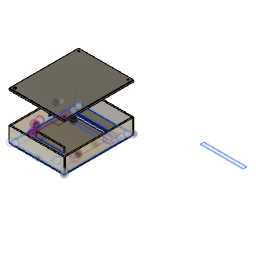
ArduinoCase v21 (Autodesk Fusion 360 design; units mm, degrees)
Autodesk Fusion 360 part; units mm, degrees
note: some values were not read from the file. Chosen so that the rebuilt part matches the saved one: which bodies a step acts on; which face or edge a step refers to; which pieces of a blend or face edit are solid. Set by a fixed rule: which sketch regions a step uses.
sketch "スケッチ1" plane through (0, 0, 0) normal (0, 0, 1) x (1, 0, 0)
  line L0 (0, 0) -> (66.06, 0)
  line L1 (68.6, 5.08) -> (68.6, 38.06)
  line L2 (64.79, 53.3) -> (0, 53.3)
  line L3 (0, 53.3) -> (0, 0)
  line L4 (64.79, 53.3) -> (68.6, 53.3)
  line L5 (68.6, 53.3) -> (68.6, 38.06)
  line L6 (66.06, 0) -> (68.6, 0)
  line L7 (68.6, 0) -> (68.6, 5.08)
  dimension "d6" = 68.6
  dimension "d7" = 53.3
  constraint horizontal L0
  constraint vertical L1
  constraint horizontal L2
  constraint vertical L3
  constraint coincident L0.start L3.end
  constraint perpendicular L1 L4
  constraint perpendicular L4 L5
  constraint perpendicular L1 L6
  constraint perpendicular L6 L7
  measures "d6" distance of L1 L3
  measures "d7" distance of L0.start L2.end
extrude "押し出し1" add sketch "スケッチ1" along normal blind 1.6 makes body 1
ref_plane "作業平面1" through (34.3, 26.65, 1.6) normal (0, 0, 1) x (1, 0, 0)
sketch "スケッチ2" plane through (34.3, 26.65, 1.6) normal (0, 0, 1) x (1, 0, 0)
  circle A0 centre (-20.33, -24.11) radius 1.6
  circle A1 centre (31.74, -19.03) radius 1.6
  circle A2 centre (31.74, 8.91) radius 1.6
  circle A3 centre (-19.06, 24.15) radius 1.6
  line L0 (-34.3, -26.65) -> (34.3, -26.65)
  line L1 (-34.3, 26.65) -> (-34.3, -26.65)
  dimension "d15" = 3.2
  dimension "d16" = 3.2
  dimension "d17" = 3.2
  dimension "d18" = 3.2
  dimension "d19" = 2.54
  dimension "d20" = 13.97
  dimension "d48" = 66.04
  dimension "d49" = 7.62
  dimension "d50" = 35.56
  dimension "d51" = 66.04
  dimension "d52" = 15.24
  dimension "d53" = 50.8
  measures "d15" diameter of A3
  measures "d16" diameter of A2
  measures "d17" diameter of A1
  measures "d18" diameter of A0
  measures "d19" distance of A0.centre L0
  measures "d20" distance of A0.centre L1
  measures "d48" distance of A1.centre L1
  measures "d49" distance of A1.centre L0
  measures "d50" distance of A2.centre L0
  measures "d51" distance of A2.centre L1
  measures "d52" distance of A3.centre L1
  measures "d53" distance of A3.centre L0
extrude "押し出し2" cut sketch "スケッチ2" against normal up to surface (1.6 mm away) bodies 1
sketch "スケッチ3" plane through (34.3, 26.65, 1.6) normal (0, 0, 1) x (1, 0, 0)
  line L0 (-36.1, -14.45) -> (-22.1, -14.45)
  line L1 (-22.1, -14.45) -> (-22.1, -23.35)
  line L2 (-22.1, -23.35) -> (-36.1, -23.35)
  line L3 (-36.1, -23.35) -> (-36.1, -14.45)
  line L4 (-34.3, 26.65) -> (-34.3, -26.65)
  line L5 (-34.3, -26.65) -> (34.3, -26.65)
  dimension "d28" = 8.9
  dimension "d29" = 14
  dimension "d30" = 1.8
  dimension "d31" = 3.3
  constraint horizontal L0
  constraint vertical L1
  constraint horizontal L2
  constraint vertical L3
  measures "d28" distance of L0.start L2.end
  measures "d29" distance of L0.start L0.end
  measures "d30" distance of L3 L4
  measures "d31" distance of L2 L5
extrude "押し出し3" add sketch "スケッチ3" along normal blind 10.9 separate body makes body 2
sketch "スケッチ4" plane through (34.3, 26.65, 1.6) normal (0, 0, 1) x (1, 0, 0)
  line L0 (-40.5, 17.05) -> (-24.5, 17.05)
  line L1 (-24.5, 17.05) -> (-24.5, 5.05)
  line L2 (-24.5, 5.05) -> (-40.5, 5.05)
  line L3 (-40.5, 5.05) -> (-40.5, 17.05)
  line L4 (34.3, 26.65) -> (-34.3, 26.65)
  line L5 (-34.3, 26.65) -> (-34.3, -26.65)
  dimension "d34" = 12
  dimension "d35" = 16
  dimension "d36" = 9.6
  dimension "d37" = 6.2
  constraint horizontal L0
  constraint vertical L1
  constraint horizontal L2
  constraint vertical L3
  measures "d34" distance of L0.start L2.end
  measures "d35" distance of L0.start L0.end
  measures "d36" distance of L0 L4
  measures "d37" distance of L3 L5
extrude "押し出し4" add sketch "スケッチ4" along normal blind 10.9 separate body makes body 3
shell "シェル1" thickness 1 removed faces 1 at (-6.2, 35.7, 5.2333) on bodies 3
ref_plane "作業平面2" through (-1.8, 7.75, 7.05) normal (-1, 0, 0) x (0, -1, 0)
sketch "スケッチ5" plane through (-1.8, 7.75, 7.05) normal (-1, 0, 0) x (0, 1, 0)
  circle A0 centre (0.05, -0.95) radius 4
  line L0 (4.45, -5.45) -> (-4.45, -5.45)
  line L1 (-4.45, 5.45) -> (-4.45, -5.45)
  dimension "d42" = 8
  dimension "d43" = 4.5
  dimension "d44" = 4.5
  measures "d42" diameter of A0
  measures "d43" distance of A0.centre L0
  measures "d44" distance of A0.centre L1
extrude "押し出し5" cut sketch "スケッチ5" against normal blind 12 bodies 2
sketch "Sketch13" plane through (0, 0, 1.6) normal (0, 0, 1) x (-1, 0, 0)
  circle A0 centre (-15.24, -50.8) radius 1.6
  circle A1 centre (-66.04, -35.56) radius 1.6
  circle A2 centre (-13.97, -2.54) radius 1.6
  circle A3 centre (-66.04, -7.62) radius 1.6
  line L0 (-68.6, -53.3) -> (0, -53.3)
  line L1 (0, -53.3) -> (0, 0)
  line L2 (0, 0) -> (-68.6, 0)
  line L3 (-68.6, 0) -> (-68.6, -53.3)
  line L4 (4.8948, -79.4441) -> (-81.6052, -79.4441)
  line L5 (-81.6052, -79.4441) -> (-81.6052, 30.5559)
  line L6 (-81.6052, 30.5559) -> (4.8948, 30.5559)
  line L7 (4.8948, 30.5559) -> (4.8948, -79.4441)
  line L8 (4.8948, -79.4441) -> (-2.1052, -79.4441)
  line L9 (-2.1052, -79.4441) -> (-2.1052, -80.4441)
  line L10 (5.8948, -72.4441) -> (4.8948, -72.4441)
  line L11 (4.8948, -72.4441) -> (4.8948, -79.4441)
  line L12 (-81.6052, -79.4441) -> (-74.6052, -79.4441)
  line L13 (-74.6052, -79.4441) -> (-74.6052, -80.4441)
  line L14 (-82.6052, -72.4441) -> (-81.6052, -72.4441)
  line L15 (-81.6052, -72.4441) -> (-81.6052, -79.4441)
  line L16 (4.8948, 30.5559) -> (-2.1052, 30.5559)
  line L17 (-2.1052, 30.5559) -> (-2.1052, 31.5559)
  line L18 (5.8948, 23.5559) -> (4.8948, 23.5559)
  line L19 (4.8948, 23.5559) -> (4.8948, 30.5559)
  line L20 (-81.6052, 30.5559) -> (-74.6052, 30.5559)
  line L21 (-74.6052, 30.5559) -> (-74.6052, 31.5559)
  line L22 (-82.6052, 23.5559) -> (-81.6052, 23.5559)
  line L23 (-81.6052, 23.5559) -> (-81.6052, 30.5559)
  arc A4 (5.8948, -72.4441) -> (-2.1052, -80.4441) centre (5.8948, -80.4441) ccw
  arc A5 (-74.6052, -80.4441) -> (-82.6052, -72.4441) centre (-82.6052, -80.4441) ccw
  arc A6 (-82.6052, 23.5559) -> (-74.6052, 31.5559) centre (-82.6052, 31.5559) ccw
  arc A7 (-2.1052, 31.5559) -> (5.8948, 23.5559) centre (5.8948, 31.5559) ccw
  line L24 (-4.5368, 3.1002) -> (-53.3368, 3.1002)
  line L25 (-53.3368, 3.1002) -> (-53.3368, 29.1002)
  line L26 (-53.3368, 29.1002) -> (-4.5368, 29.1002)
  line L27 (-4.5368, 29.1002) -> (-4.5368, 3.1002)
  line L28 (-53.3368, 3.1002) -> (-8.3368, 3.1002)
  line L29 (-8.3368, 3.1002) -> (-8.3368, 1.1002)
  line L30 (-8.3368, 1.1002) -> (-53.3368, 1.1002)
  line L31 (-53.3368, 1.1002) -> (-53.3368, 3.1002)
  line L32 (-152.4076, -126.3216) -> (-222.4076, -126.3216)
  line L33 (-222.4076, -126.3216) -> (-222.4076, -122.3216)
  line L34 (-222.4076, -122.3216) -> (-152.4076, -122.3216)
  line L35 (-152.4076, -122.3216) -> (-152.4076, -126.3216)
  circle A8 centre (2.0051, -76.5556) radius 1.85
  circle A9 centre (-78.6355, -76.6374) radius 1.85
  circle A10 centre (-78.6896, 27.6935) radius 1.85
  circle A11 centre (2.0228, 27.6497) radius 1.85
  circle A12 centre (-15.24, -50.8) radius 2.5
  circle A13 centre (-66.04, -7.62) radius 2.5
  line L36 (1.0324, -67.1894) -> (-78.9676, -67.1894)
  line L37 (-78.9676, -67.1894) -> (-78.9676, -47.1894)
  line L38 (-78.9676, -47.1894) -> (1.0324, -47.1894)
  line L39 (1.0324, -47.1894) -> (1.0324, -67.1894)
  line L40 (-72.9759, 3.4319) -> (-72.9759, 21.4319)
  line L41 (-72.9759, 21.4319) -> (-54.9759, 21.4319)
  line L42 (-54.9759, 21.4319) -> (-54.9759, 3.4319)
  line L43 (-54.9759, 3.4319) -> (-72.9759, 3.4319)
  circle A14 centre (-57.4759, 18.9319) radius 2.5
  line L44 (-81.6052, -79.4441) -> (-83.6052, -79.4441)
  line L45 (-83.6052, -79.4441) -> (-83.6052, 30.5559)
  line L46 (-83.6052, 30.5559) -> (-81.6052, 30.5559)
  line L47 (-81.6052, 30.5559) -> (-81.6052, -79.4441)
  line L48 (4.8948, -79.4441) -> (6.8948, -79.4441)
  line L49 (6.8948, -79.4441) -> (6.8948, 30.5559)
  line L50 (6.8948, 30.5559) -> (4.8948, 30.5559)
  line L51 (4.8948, 30.5559) -> (4.8948, -79.4441)
  line L52 (6.8948, 30.5559) -> (-83.6176, 30.5559)
  line L53 (-83.6176, 30.5559) -> (-83.6176, 32.5559)
  line L54 (-83.6176, 32.5559) -> (6.8948, 32.5559)
  line L55 (6.8948, 32.5559) -> (6.8948, 30.5559)
  line L56 (6.8948, -79.4441) -> (-83.6077, -79.4441)
  line L57 (-83.6077, -79.4441) -> (-83.6077, -81.4441)
  line L58 (-83.6077, -81.4441) -> (6.8948, -81.4441)
  line L59 (6.8948, -81.4441) -> (6.8948, -79.4441)
  circle A15 centre (-78.6896, 27.6935) radius 2.5
  circle A16 centre (2.0228, 27.6497) radius 2.5
  circle A17 centre (2.0051, -76.5556) radius 2.5
  circle A18 centre (-78.6355, -76.6374) radius 2.5
  circle A19 centre (-38.8293, 30.5559) radius 1.0555
  line L60 (1.0324, -47.1894) -> (-78.9676, -47.1894)
  line L61 (-78.9676, -47.1894) -> (-78.9676, -53.1894)
  line L62 (-78.9676, -53.1894) -> (1.0324, -53.1894)
  line L63 (1.0324, -53.1894) -> (1.0324, -47.1894)
  line L64 (1.0324, -67.1894) -> (-78.9676, -67.1894)
  line L65 (-78.9676, -67.1894) -> (-78.9676, -61.1894)
  line L66 (-78.9676, -61.1894) -> (1.0324, -61.1894)
  line L67 (1.0324, -61.1894) -> (1.0324, -67.1894)
  line L68 (-152.4075, -127.8529) -> (-222.4075, -127.8529)
  line L69 (-222.4075, -127.8529) -> (-222.4075, -120.8529)
  line L70 (-222.4075, -120.8529) -> (-152.4075, -120.8529)
  line L71 (-152.4075, -120.8529) -> (-152.4075, -127.8529)
  line L72 (-4.0011, -64.7327) -> (-74.0011, -64.7327)
  line L73 (-74.0011, -64.7327) -> (-74.0011, -57.7327)
  line L74 (-74.0011, -57.7327) -> (-4.0011, -57.7327)
  line L75 (-4.0011, -57.7327) -> (-4.0011, -64.7327)
  line L76 (-4.0011, -63.2327) -> (-74.0011, -63.2327)
  line L77 (-74.0011, -63.2327) -> (-74.0011, -59.2327)
  line L78 (-74.0011, -59.2327) -> (-4.0011, -59.2327)
  line L79 (-4.0011, -59.2327) -> (-4.0011, -63.2327)
  line L80 (-78.9855, -67.1473) -> (-73.9855, -67.1473)
  line L81 (-73.9855, -67.1473) -> (-73.9855, -61.1473)
  line L82 (-73.9855, -61.1473) -> (-78.9855, -61.1473)
  line L83 (-78.9855, -61.1473) -> (-78.9855, -67.1473)
  line L84 (-78.9676, -47.1894) -> (-65.9676, -47.1894)
  line L85 (-65.9676, -47.1894) -> (-65.9676, -53.1894)
  line L86 (-65.9676, -53.1894) -> (-78.9676, -53.1894)
  line L87 (-78.9676, -53.1894) -> (-78.9676, -47.1894)
  circle A20 centre (0.015, -66.0578) radius 2.5
  circle A21 centre (-78.1357, -66.0415) radius 2.5
  circle A22 centre (-66.04, -7.62) radius 0.725
  circle A23 centre (-15.24, -50.8) radius 0.725
  circle A24 centre (0.015, -66.0578) radius 0.725
  circle A25 centre (-78.1357, -66.0415) radius 0.725
  circle A26 centre (-57.4759, 18.9319) radius 0.725
  line L88 (6.8948, -81.4441) -> (-83.6176, -81.4441)
  line L89 (-83.6176, -81.4441) -> (-83.6176, 32.5559)
  line L90 (-83.6176, 32.5559) -> (6.8948, 32.5559)
  line L91 (6.8948, 32.5559) -> (6.8948, -81.4441)
  point P0 (6.8948, -81.4441)
  point P1 (-83.6077, -81.4441)
  point P2 (-83.6176, 32.5559)
  dimension "d96" = 7
  dimension "d97" = 7
  dimension "d98" = 7
  dimension "d99" = 7
  dimension "d100" = 7
  dimension "d101" = 7
  dimension "d102" = 7
  dimension "d103" = 7
  dimension "d104" = 8
  dimension "d105" = 48.8
  dimension "d106" = 26
  dimension "d107" = 45
  dimension "d108" = 2
  dimension "d116" = 70
  dimension "d117" = 4
  dimension "d118" = 3.7
  dimension "d119" = 3.7
  dimension "d120" = 3.7
  dimension "d121" = 3.7
  dimension "d122" = 5
  dimension "d123" = 5
  dimension "d124" = 80
  dimension "d125" = 20
  dimension "d126" = 18
  dimension "d127" = 18
  dimension "d128" = 5
  dimension "d129" = 110
  dimension "d130" = 86.5
  dimension "d131" = 2
  dimension "d132" = 2
  dimension "d133" = 2
  dimension "d134" = 2
  dimension "d135" = 5
  dimension "d137" = 5
  dimension "d138" = 5
  dimension "d139" = 5
  dimension "d140" = 6
  dimension "d141" = 6
  dimension "d142" = 70
  dimension "d143" = 7
  dimension "d151" = 70
  dimension "d152" = 7
  dimension "d153" = 70
  dimension "d154" = 4
  dimension "d155" = 5
  dimension "d156" = 6
  dimension "d157" = 6
  dimension "d158" = 13
  dimension "d159" = 5
  dimension "d160" = 5
  dimension "d169" = 1.45
  dimension "d170" = 1.45
  dimension "d171" = 1.45
  dimension "d172" = 1.45
  dimension "d173" = 1.45
  constraint horizontal L4
  constraint vertical L5
  constraint horizontal L6
  constraint vertical L7
  constraint horizontal L8
  constraint vertical L9
  constraint horizontal L10
  constraint vertical L11
  constraint horizontal L12
  constraint vertical L13
  constraint horizontal L14
  constraint vertical L15
  constraint horizontal L16
  constraint vertical L17
  constraint horizontal L18
  constraint vertical L19
  constraint horizontal L20
  constraint vertical L21
  constraint horizontal L22
  constraint vertical L23
  constraint tangent L9 A4
  constraint tangent L10 A4
  constraint tangent L13 A5
  constraint tangent L14 A5
  constraint equal A4 A5
  constraint tangent L22 A6
  constraint tangent L21 A6
  constraint equal A4 A6
  constraint tangent L18 A7
  constraint tangent L17 A7
  constraint equal A4 A7
  constraint horizontal L24
  constraint vertical L25
  constraint horizontal L26
  constraint vertical L27
  constraint horizontal L28
  constraint vertical L29
  constraint horizontal L30
  constraint vertical L31
  constraint horizontal L32
  constraint vertical L33
  constraint horizontal L34
  constraint vertical L35
  constraint concentric A0 A12
  constraint concentric A3 A13
  constraint horizontal L36
  constraint vertical L37
  constraint horizontal L38
  constraint vertical L39
  constraint tangent L42 A14
  constraint tangent L41 A14
  constraint horizontal L44
  constraint vertical L45
  constraint horizontal L46
  constraint vertical L47
  constraint equal L5 L45
  constraint horizontal L48
  constraint vertical L49
  constraint horizontal L50
  constraint vertical L51
  constraint equal L7 L49
  constraint horizontal L52
  constraint vertical L53
  constraint horizontal L54
  constraint vertical L55
  constraint horizontal L56
  constraint vertical L57
  constraint horizontal L58
  constraint vertical L59
  constraint concentric A10 A15
  constraint tangent A6 A15
  constraint concentric A11 A16
  constraint tangent A7 A16
  constraint concentric A8 A17
  constraint tangent A4 A17
  constraint concentric A9 A18
  constraint tangent A5 A18
  constraint coincident L52 A19.centre
  constraint horizontal L60
  constraint vertical L61
  constraint horizontal L62
  constraint vertical L63
  constraint horizontal L64
  constraint vertical L65
  constraint horizontal L66
  constraint vertical L67
  constraint horizontal L68
  constraint vertical L69
  constraint horizontal L70
  constraint vertical L71
  constraint horizontal L72
  constraint vertical L73
  constraint horizontal L74
  constraint vertical L75
  constraint horizontal L76
  constraint vertical L77
  constraint horizontal L78
  constraint vertical L79
  constraint midpoint L75 L79
  constraint horizontal L80
  constraint vertical L81
  constraint horizontal L82
  constraint vertical L83
  constraint horizontal L84
  constraint vertical L85
  constraint horizontal L86
  constraint vertical L87
  constraint concentric A13 A22
  constraint concentric A12 A23
  constraint concentric A20 A24
  constraint concentric A21 A25
  constraint concentric A14 A26
  constraint coincident P0 L58.end
  constraint coincident P1 L57.end
  constraint coincident P2 L53.end
  constraint horizontal L88
  constraint vertical L89
  constraint horizontal L90
  constraint vertical L91
  measures "d96" distance of L4.start L8.end
  measures "d97" distance of L4.start L10.end
  measures "d98" distance of L4.end L12.end
  measures "d99" distance of L4.end L14.end
  measures "d100" distance of L6.end L16.end
  measures "d101" distance of L6.end L18.end
  measures "d102" distance of L5.end L20.end
  measures "d103" distance of L5.end L22.end
  measures "d104" radius of A4
  measures "d105" distance of L24.start L24.end
  measures "d106" distance of L24.start L26.end
  measures "d107" distance of L24.end L28.end
  measures "d108" distance of L24.end L30.end
  measures "d116" distance of L32.start L32.end
  measures "d117" distance of L32.start L34.end
  measures "d118" diameter of A8
  measures "d119" diameter of A9
  measures "d120" diameter of A10
  measures "d121" diameter of A11
  measures "d122" diameter of A12
  measures "d123" diameter of A13
  measures "d124" distance of L36.start L36.end
  measures "d125" distance of L36.start L38.end
  measures "d126" distance of L40.start L40.end
  measures "d127" distance of L40.start L42.end
  measures "d128" diameter of A14
  measures "d129" distance of L4.end L5.end
  measures "d130" distance of L5.end L6.end
  measures "d131" distance of L4.start L48.end
  measures "d132" distance of L4.end L44.end
  measures "d133" distance of L52.end P2
  measures "d134" distance of L48.end L58
  measures "d135" diameter of A15
  measures "d137" diameter of A16
  measures "d138" diameter of A17
  measures "d139" diameter of A18
  measures "d140" distance of L38.end L62.end
  measures "d141" distance of L36.start L66.end
  measures "d142" distance of L68.start L68.end
  measures "d143" distance of L68.start L70.end
  measures "d151" distance of L72.start L72.end
  measures "d152" distance of L72.start L74.end
  measures "d153" distance of L76.start L76.end
  measures "d154" distance of L76.start L78.end
  measures "d155" distance of L80.start L80.end
  measures "d156" distance of L80.start L82.end
  measures "d157" distance of L37.end L61.end
  measures "d158" distance of L37.end L84.end
  measures "d159" diameter of A20
  measures "d160" diameter of A21
  measures "d169" diameter of A22
  measures "d170" diameter of A23
  measures "d171" diameter of A24
  measures "d172" diameter of A25
  measures "d173" diameter of A26
extrude "Extrude6" add sketch "Sketch13" along normal blind 24 and the other way blind 0 contours L4 L8 L9 L12 L13 A4 A5 L44 L48 L56 L57 L58 L59 L88 L91 | L4 L8 L9 A4 L56 | L4 L12 L13 A5 L56 | L7 L10 L11 L18 L19 A4 A7 L48 L49 L50 L51 L52 L56 L91 | L5 L14 L15 L22 L23 A5 A6 L44 L45 L46 L47 L52 L56 | L7 L10 L11 A4 L51 | L5 L14 L15 A5 L47 | L6 L16 L17 L20 L21 A6 A7 L46 L50 L52 L53 L54 L55 A19 L89 L90 L91 | L7 L18 L19 A7 L51 | L5 L22 L23 A6 L47 | L6 L16 L17 A7 L52 | L6 L20 L21 A6 L52 | L6 L52 A19 picked at (-38.6534, 30.8605) bodies 3
extrude "Extrude7" add sketch "Sketch13" along normal blind 8 contours L6 L52 A19 | L6 L52 A19 | L24 L28 L29 L30 L31 bodies 3 makes body 4 at (23.3368, -1.1002, 4.2667)
extrude "Extrude8" add sketch "Sketch13" along normal blind 3.56 contours A17 | L4 L7 L8 L11 A4 L51 L56 | A18 | L4 L5 L12 L15 A5 L47 L56 | A16 | L6 L7 L16 L19 A7 L51 L52 | A15 | L5 L6 L20 L23 A6 L47 L52 bodies 3
extrude "Extrude9" add sketch "Sketch13" along normal blind 4 separate body contours A0 | A3 | A12 L62 | A13 | A14 picked at (-15.2799, -52.9248) makes body 5 at (57.7209, -16.444, 4.2667) makes body 6 at (63.5524, 7.8689, 4.2667) makes body 7 at (16.4271, 53.0002, 4.2667)
move_body "Move1" bodies 2 1 to x (1, 0, 0) y (0, 1, 0) z (0, 0, 1) at (0, 0, 5.75)
extrude "Extrude10" add sketch "Sketch13" along normal blind 17 separate body contours L37 L65 L80 A21 | L36 L37 L64 L65 L80 L83 A21 | L36 L39 L64 L67 A20 | L36 L39 L64 L67 A20 makes body 8 at (75.6914, 66.5663, 12.9333) makes body 8 at (75.9748, 67.2986, 12.9333) makes body 9 at (2.3343, 65.2028, 12.9333)
sketch "Sketch14" plane through (-6.8948, 0, 0) normal (-1, 0, 0) x (0, -1, 0)
  line L0 (-81.4441, 1.6) -> (32.5559, 1.6)
  line L1 (32.5559, 1.6) -> (32.5559, 25.6)
  line L2 (32.5559, 25.6) -> (-81.4441, 25.6)
  line L3 (-81.4441, 25.6) -> (-81.4441, 1.6)
  line L4 (-44.1664, 19.2577) -> (-31.1664, 19.2577)
  line L5 (-31.1664, 19.2577) -> (-31.1664, 7.2577)
  line L6 (-31.1664, 7.2577) -> (-44.1664, 7.2577)
  line L7 (-44.1664, 7.2577) -> (-44.1664, 19.2577)
  dimension "d178" = 13
  dimension "d179" = 12
  constraint horizontal L4
  constraint vertical L5
  constraint horizontal L6
  constraint vertical L7
  measures "d178" distance of L4.start L4.end
  measures "d179" distance of L4.start L6.end
extrude "Extrude11" cut sketch "Sketch14" against normal blind 4 contours L4 L5 L6 L7 bodies 3
delete_face "DeleteFace1" 1 faces at (5.5684, 43.7, 7.1192) on bodies 3
chamfer "Chamfer1" distance 0.25 angle 45 4 edges at (-6.8948, 37.6664, 7.2577) (-6.8948, 31.1664, 13.2577) (-6.8948, 37.6664, 19.2577) (-6.8948, 44.1664, 13.2577) on bodies 3
sketch "Sketch15" plane through (0, 0, 1.6) normal (0, 0, 1) x (-1, 0, 0)
box "BoxPrimitive1" add length 113.9984 width 90.5019 height 2 placed x (0, 1, 0) y (-1, 0, 0) z (0, 0, 1) at (83.6075, -32.5547, 1.6) separate body makes body 10
move_body "Move2" bodies 10 to x (1, 0, 0) y (0, 1, 0) z (0, 0, 1) at (0, 0, -1.9)
sketch "Sketch21" plane through (0, 0, 0) normal (0, 0, 1) x (1, 0, 0)
  line L0 (-6.8952, 81.4441) -> (83.6169, 81.4441)
  line L1 (83.6169, 81.4441) -> (83.6169, -32.5558)
  line L2 (83.6169, -32.5558) -> (-6.8952, -32.5558)
  line L3 (-6.8952, -32.5558) -> (-6.8952, 81.4441)
  circle A0 centre (78.6819, -27.6823) radius 0.75
  circle A1 centre (-2.0299, -27.6823) radius 1.5
  circle A2 centre (-2.0299, 76.565) radius 0.75
  circle A3 centre (78.6205, 76.6443) radius 0.75
  dimension "d214" = 1.5
  dimension "d215" = 1.5
  dimension "d216" = 3
  dimension "d217" = 1.5
  constraint horizontal L0
  constraint vertical L1
  constraint horizontal L2
  constraint vertical L3
  measures "d214" diameter of A3
  measures "d215" diameter of A2
  measures "d216" diameter of A1
  measures "d217" diameter of A0
extrude "Extrude16" add sketch "Sketch21" along normal blind 2 separate body makes body 11
move_body "Move3" bodies 11 to x (1, 0, 0) y (0, 1, 0) z (0, 0, 1) at (0, 0, 40)
move_face "MoveFace1" by (0, 0, 1) 1 faces at (51.7462, 7.5005, 42) on bodies 11
chamfer "Chamfer2" distance 0.5 angle 45 4 edges at (38.3608, -32.5558, 43) (83.6169, 24.4442, 43) (-6.8952, 24.4442, 43) (38.3608, 81.4441, 43) on bodies 11
fillet "Fillet2" radius 0.5 4 edges at (-6.6452, 81.1941, 42.75) (83.3669, 81.1941, 42.75) (83.3669, -32.3058, 42.75) (-6.6452, -32.3058, 42.75) on bodies 11
move_body "Move4" bodies 11 to x (1, 0, 0) y (0, 1, 0) z (0, 0, 1) at (0, 0, 20)
extrude "Extrude12" cut sketch "Sketch13" along normal blind 3 contours L66 L73 L75 L77 L78 L79 L81 L82 | L66 L75 L76 L79 L81 bodies 10
extrude "Extrude13" cut sketch "Sketch13" against normal blind 4 contours L66 L73 L75 L77 L78 L79 L81 L82 | L66 L75 L76 L79 L81 bodies 10
extrude "Extrude14" cut sketch "Sketch13" against normal blind 1 contours L73 L74 L75 L78 | L72 L75 L76 L81 bodies 10
extrude "Extrude15" cut sketch "Sketch13" along normal blind 2 contours L73 L74 L75 L78 | L72 L75 L76 L81 bodies 10
extrude "Extrude17" cut sketch "Sketch21" against normal blind 15 contours A0 | A1 | A2 | A3 bodies 10
extrude "Extrude18" cut sketch "Sketch13" against normal blind 5 contours A8 | A9 | A10 | A11 bodies 10
extrude "Extrude19" cut sketch "Sketch13" along normal blind 25 contours A8 | A9 | A10 | A11 bodies 10
chamfer "Chamfer3" distance 0.5 angle 45 4 edges at (-3.4284, -27.1399, 63) (77.9827, -27.4111, 63) (77.9213, 76.9155, 63) (-2.7292, 76.8362, 63) on bodies 11
chamfer "Chamfer5" distance 0.75 angle 45 4 edges at (-6.8944, 24.4445, -0.3) (38.3565, -32.5547, -0.3) (38.3565, 81.4437, -0.3) (83.6075, 24.4445, -0.3) on bodies 10
chamfer "Chamfer4" distance 0.3 angle 45 12 edges at (-6.8948, 81.4441, 13.6) (83.6077, 81.4441, 13.6) (83.6176, -32.5559, 13.6) (-6.8948, -32.5559, 13.6) (-6.8952, 81.4441, 61.2026) (83.6169, 81.4441, 61.2026) (83.6169, -32.5558, 61.2026) (-6.8952, -32.5558, 61.2026) (-6.8944, 81.4437, 0.7) (83.6075, 81.4437, 0.7) (83.6075, -32.5547, 0.7) (-6.8944, -32.5547, 0.7) on bodies 3 10 11
sketch "Sketch22" plane through (-6.8948, 0, 0) normal (-1, 0, 0) x (0, -1, 0)
  line L0 (32.2559, 1.6) -> (32.2559, 25.6)
  line L1 (32.2559, 25.6) -> (-81.1441, 25.6)
  line L2 (-81.1441, 25.6) -> (-81.1441, 1.6)
  line L3 (-81.1441, 1.6) -> (32.2559, 1.6)
  line L4 (-44.4164, 19.5077) -> (-30.9164, 19.5077)
  line L5 (-30.9164, 19.5077) -> (-30.9164, 7.0077)
  line L6 (-30.9164, 7.0077) -> (-44.4164, 7.0077)
  line L7 (-44.4164, 7.0077) -> (-44.4164, 19.5077)
  line L8 (-76.8733, -0.2812) -> (-75.9434, -0.2812)
  line L9 (-75.9434, -0.2812) -> (-75.9434, 27.2267)
  line L10 (-75.9434, 27.2267) -> (-76.8733, 27.2267)
  line L11 (-76.8733, 27.2267) -> (-76.8733, -0.2812)
  constraint horizontal L8
  constraint vertical L9
  constraint horizontal L10
  constraint vertical L11
sketch "Sketch23" plane through (-6.8948, 0, 0) normal (-1, 0, 0) x (0, -1, 0)
  line L0 (32.2559, 1.6) -> (32.2559, 25.6)
  line L1 (32.2559, 25.6) -> (-81.1441, 25.6)
  line L2 (-81.1441, 25.6) -> (-81.1441, 1.6)
  line L3 (-81.1441, 1.6) -> (32.2559, 1.6)
  line L4 (-44.4164, 19.5077) -> (-30.9164, 19.5077)
  line L5 (-30.9164, 19.5077) -> (-30.9164, 7.0077)
  line L6 (-30.9164, 7.0077) -> (-44.4164, 7.0077)
  line L7 (-44.4164, 7.0077) -> (-44.4164, 19.5077)
  line L8 (-44.4164, 19.5077) -> (-52.4164, 19.5077)
  line L9 (-52.4164, 19.5077) -> (-52.4164, 22.6279)
  line L10 (-52.4164, 22.6279) -> (-44.4164, 22.6279)
  line L11 (-44.4164, 22.6279) -> (-44.4164, 19.5077)
  circle A0 centre (-52.4098, 17.788) radius 1.25
  dimension "d209" = 8
  dimension "d210" = 2.5
  constraint horizontal L8
  constraint vertical L9
  constraint horizontal L10
  constraint vertical L11
  constraint coincident L4.start L7.end
  measures "d209" distance of L4.start L8.end
  measures "d210" diameter of A0
extrude "Extrude20" cut sketch "Sketch23" against normal blind 3 contours A0 bodies 3
chamfer "Chamfer6" distance 0.25 angle 45 2 edges at (-6.8948, 53.5752, 18.24) (-4.8948, 53.5752, 17.336) on bodies 3
move_body "Move5" bodies 11 to x (1, 0, 0) y (0, 1, 0) z (0, 0, 1) at (0, 0.0486, -34.3877)
move_body "Move6" bodies 11 to x (1, 0, 0) y (0, 1, 0) z (0, 0, 1) at (0, 0, 50)
sketch "Sketch26" plane through (0, 0, -0.3) normal (0, 0, -1) x (1, 0, 0)
  line L0 (73.9855, -63.2327) -> (4.0011, -63.2327)
  line L1 (4.0011, -63.2327) -> (4.0011, -59.2327)
  line L2 (4.0011, -59.2327) -> (74.0011, -59.2327)
  line L3 (74.0011, -59.2327) -> (74.0011, -61.1473)
  line L4 (74.0011, -61.1473) -> (73.9855, -61.1473)
  line L5 (73.9855, -61.1473) -> (73.9855, -63.2327)
  circle A0 centre (78.6355, -76.6374) radius 1.85
  circle A1 centre (-2.0051, -76.5556) radius 1.85
  circle A2 centre (78.6896, 27.6935) radius 1.85
  circle A3 centre (-2.0228, 27.6497) radius 1.85
  line L6 (82.8575, -80.6937) -> (82.8575, 31.8047)
  line L7 (82.8575, 31.8047) -> (-6.1444, 31.8047)
  line L8 (-6.1444, 31.8047) -> (-6.1444, -80.6937)
  line L9 (-6.1444, -80.6937) -> (82.8575, -80.6937)
hidden bodies 1 2
named bodies: "body", "dc_plug", "sidewalls", "battery wall", "screwholes (2)", "screwholes (1)", "screwholes", "ScrewHoles (1)", "ScrewHoles", "Bottom Piece", "Top Lid"
